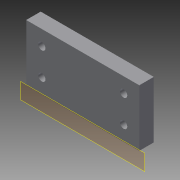
# Autodesk Inventor part: basePlate01
Saved by Autodesk Inventor 2013 (Build 170138000, 138)
## iProperties
Created: 2013-02-22
Part Number: basePlate01
Material: Generic
Document SubType Name: Modeling
Designer: Nano
Density: 1 g/cm^3
Author: Nano
Autodesk Inventor part; units mm, degrees
ref_plane "YZ Plane" through (0, 0, 0) normal (1, 0, 0) x (0, 1, 0)
ref_plane "XZ Plane" through (0, 0, 0) normal (0, 1, 0) x (-1, 0, 0)
ref_plane "XY Plane" through (0, 0, 0) normal (0, 0, 1) x (1, 0, 0)
ref_plane "Work Plane1" through (0, 0, 0) normal (0, 0, 1) x (1, 0, 0)
sketch "Sketch1" plane through (0, 0, 0) normal (0, 0, 1) x (1, 0, 0)
  line L0 (-17.7099, -6.35) -> (57.15, -6.35) projected
  line L1 (57.15, 0) -> (-17.7099, 0) projected
  line L2 (1.3284, -28.575) -> (1.3284, 22.225) projected
  line L3 (1.3284, -28.575) -> (7.6784, -28.575) projected
  line L4 (7.6784, 22.225) -> (7.6784, -28.575) projected
  line L5 (1.3284, 22.225) -> (7.6784, 22.225) projected
  line L6 (63.5, -28.575) -> (63.5, 22.225) projected
  line L7 (63.5, 22.225) -> (57.15, 22.225) projected
  line L8 (57.15, -28.575) -> (57.15, 22.225) projected
  line L9 (63.5, -28.575) -> (57.15, -28.575) projected
  line L10 (7.6835, 0) -> (57.15, 0)
  line L11 (57.15, 0) -> (57.15, 22.225)
  line L12 (57.15, 22.225) -> (7.6835, 22.225)
  line L13 (7.6835, 22.225) -> (7.6835, 0)
  circle A0 centre (14.5257, 3.9217) radius 1.5875
  line L14 (32.4168, 24.8107) -> (32.4168, 0) construction
  circle A1 centre (50.3079, 3.9217) radius 1.5875
  line L15 (7.6835, 11.1125) -> (57.15, 11.1125) construction
  circle A2 centre (14.5257, 18.3033) radius 1.5875
  circle A3 centre (50.3079, 18.3033) radius 1.5875
  line L16 (57.15, 0) -> (57.15, -6.35) projected
  line L17 (-17.7099, 0) -> (-17.7099, -6.35) projected
  line L18 (57.15, 0) -> (63.5, 0) projected
  point P0 (0, 0)
  dimension "d0" = 3.175
  dimension "d3" = 22.225
  dimension "d4" = 11.1125
  constraints: 12 end point, 4 centre point, 3 symmetric about line, 2 parallel, 1 horizontal, 1 perpendicular, 3 other
  measures "d0" diameter of A0
  measures "d3" distance of L11.end L1.start
  measures "d4" distance between parallel lines of L10 L15
extrude "Extrusion1" add sketch "Sketch1" against normal blind 6.35 contours L1 L13 L12 L8
equation "\"d4\" = 0.5 * d3"
body "Solid1"
